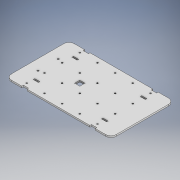
# Autodesk Inventor part: FPVchasisdraft2
Saved by Autodesk Inventor 2020 (Build 240168000, 168)
## iProperties
Created: 2020-11-26
Part Number: FPVchasisdraft2
Material: Generic
Document SubType Name: Modeling
Designer: yeyet
Density: 1 g/cm^3
Appearance: Default
Author: yeyet
Autodesk Inventor part; units mm, degrees
sketch "Sketch1" plane through (0, 0, 0) normal (0, 0, 1) x (1, 0, 0)
  line L0 (0, 0) -> (200, 0)
  line L1 (200, 0) -> (200, 120)
  line L2 (200, 120) -> (0, 120)
  line L3 (0, 120) -> (0, 0)
  dimension "d6" = 200
  dimension "d7" = 120
  constraints: 8 end point, 2 parallel, 1 horizontal, 1 perpendicular
  measures "d6" distance of L1.end L2.end
  measures "d7" distance of L0.end L1.end
extrude "Extrusion1" add sketch "Sketch1" along normal blind 3
sketch "Sketch2" plane through (0, 0, 3) normal (0, 0, 1) x (1, 0, 0)
  line L0 (0, 120) -> (0, 0) construction
  line L1 (0, 60) -> (200, 60) construction
  line L2 (200, 0) -> (200, 120) construction
  line L3 (200, 120) -> (0, 120) construction
  line L4 (100, 120) -> (100, 0) construction
  line L5 (0, 0) -> (200, 0) construction
  point P0 (30, 43.15)
  dimension "d10" = 16.85
  dimension "d11" = 30
  constraints: 4 end point, 4 midpoint
  measures "d10" distance from line of L1 point (30, 43.15)
  measures "d11" distance from line of point (30, 43.15) L0
hole "Hole1" at (30, 43.15, 3) direction (0, 0, -1) diameter 2.85 end through all thread size "M3.5x0.6" class "6H" standard "ISO Metric profile"
ref_plane "Work Plane1" through (0, 60, 0) normal (0, 1, 0) x (1, 0, 0)
mirror "Mirror1" about plane through (0, 60, 0) normal (0, 1, 0) of "Hole1"
pattern_linear "Rectangular Pattern1" count 2 spacing 33.7 along (1, 0, 0) of "Hole1", "Mirror1"
pattern_linear "Rectangular Pattern2" count 4 spacing 33.7 along (1, 0, 0) count 2 spacing 33.7 along (0, 1, 0) of "Hole1", "Mirror1", "Rectangular Pattern1"
mirror "Mirror2" about plane through (0, 60, 0) normal (0, 1, 0) of "Hole1", "Mirror1", "Rectangular Pattern1", "Rectangular Pattern2"
sketch "Sketch3" plane through (0, 0, 3) normal (0, 0, 1) x (1, 0, 0)
  line L0 (75.55, 65) -> (85.55, 65)
  line L1 (85.55, 65) -> (85.55, 55)
  line L2 (85.55, 55) -> (75.55, 55)
  line L3 (75.55, 55) -> (75.55, 65)
  circle A0 centre (63.7, 76.85) radius 1.425 construction
  circle A1 centre (97.4, 43.15) radius 1.425 construction
  line L4 (63.7, 76.85) -> (97.4, 43.15) construction
  circle A2 centre (97.4, 76.85) radius 1.425 construction
  circle A3 centre (63.7, 43.15) radius 1.425 construction
  line L5 (63.7, 43.15) -> (97.4, 76.85) construction
  point P0 (0, 0)
  point P1 (80.55, 65)
  point P2 (80.55, 60)
  point P3 (85.55, 60)
  point P4 (80.55, 60)
  dimension "d28" = 10
  dimension "d29" = 10
  constraints: 12 end point, 4 midpoint, 2 parallel, 1 horizontal, 1 horizontal alignment, 1 perpendicular, 1 vertical alignment
  measures "d28" distance of L0.end L1.end
  measures "d29" distance of L0.start L0.end
extrude "Extrusion2" cut sketch "Sketch3" against normal through all
sketch "Sketch4" plane through (0, 0, 3) normal (0, 0, 1) x (1, 0, 0)
  line L0 (0, 0) -> (200, 0) construction
  line L1 (30, 0) -> (40, 0)
  line L2 (40, 0) -> (40, 3)
  line L3 (40, 3) -> (30, 3)
  line L4 (30, 3) -> (30, 0)
  line L5 (0, 120) -> (0, 0) construction
  line L6 (30, 24.6) -> (40, 24.6)
  line L7 (40, 24.6) -> (40, 21.6)
  line L8 (40, 21.6) -> (30, 21.6)
  line L9 (30, 21.6) -> (30, 24.6)
  dimension "d32" = 3
  dimension "d33" = 10
  dimension "d34" = 30
  dimension "d35" = 18.6
  dimension "d36" = 3
  dimension "d37" = 10
  constraints: 16 end point, 4 parallel, 2 horizontal, 2 perpendicular, 2 point on line
  measures "d32" distance of L3.end L1.start
  measures "d33" distance of L2.end L3.end
  measures "d34" distance between parallel lines of L5 L4
  measures "d35" distance between parallel lines of L3 L8
  measures "d36" distance of L6.end L7.end
  measures "d37" distance of L6.start L6.end
extrude "Extrusion3" cut sketch "Sketch4" against normal through all
ref_plane "Work Plane66" through (0, 60, 0) normal (0, 1, 0) x (1, 0, 0)
mirror "Mirror3" about plane through (0, 60, 0) normal (0, 1, 0) of "Extrusion3"
ref_plane "Work Plane67" through (100, 0, 0) normal (-1, 0, 0) x (0, 0, 1)
mirror "Mirror4" about plane through (100, 0, 0) normal (-1, 0, 0) of "Extrusion3", "Mirror3"
sketch "Sketch5" plane through (0, 0, 3) normal (0, 0, 1) x (1, 0, 0)
  line L0 (0, 120) -> (0, 0) construction
  line L1 (0, 120) -> (0, 0) construction
  line L2 (0, 60) -> (200, 60) construction
  line L3 (200, 0) -> (200, 120) construction
  point P0 (20, 40.7)
  dimension "d40" = 20
  dimension "d41" = 19.3
  constraints: 2 end point, 2 midpoint
  measures "d40" distance from line of point (20, 40.7) L0
  measures "d41" distance from line of L2 point (20, 40.7)
hole "Hole2" at (20, 40.7, 3) direction (0, 0, -1) diameter 3.242 end through all thread size "M4x0.7" class "6H" standard "ISO Metric profile"
ref_plane "Work Plane68" through (40, 60, 0) normal (0, -1, 0) x (1, 0, 0)
mirror "Mirror5" about plane through (40, 60, 0) normal (0, -1, 0) of "Hole2"
fillet "Fillet1" radius 10 4 edges at (0, 120, 1.5) (0, 0, 1.5) (200, 0, 1.5) (200, 120, 1.5)
ref_plane "Work Plane2" through (0, 60, 0) normal (0, 1, 0) x (1, 0, 0)
ref_plane "Work Plane4" through (33.7, 60, 0) normal (0, 1, 0) x (1, 0, 0)
ref_plane "Work Plane5" through (33.7, 60, 0) normal (0, 1, 0) x (1, 0, 0)
ref_plane "Work Plane6" through (33.7, 60, 0) normal (0, 1, 0) x (1, 0, 0)
ref_plane "Work Plane7" through (67.4, 60, 0) normal (0, 1, 0) x (1, 0, 0)
ref_plane "Work Plane8" through (101.1, 60, 0) normal (0, 1, 0) x (1, 0, 0)
ref_plane "Work Plane9" through (0, 93.7, 0) normal (0, 1, 0) x (1, 0, 0)
ref_plane "Work Plane10" through (33.7, 93.7, 0) normal (0, 1, 0) x (1, 0, 0)
ref_plane "Work Plane11" through (67.4, 93.7, 0) normal (0, 1, 0) x (1, 0, 0)
ref_plane "Work Plane12" through (101.1, 93.7, 0) normal (0, 1, 0) x (1, 0, 0)
ref_plane "Work Plane13" through (33.7, 60, 0) normal (0, 1, 0) x (1, 0, 0)
ref_plane "Work Plane14" through (67.4, 60, 0) normal (0, 1, 0) x (1, 0, 0)
ref_plane "Work Plane15" through (101.1, 60, 0) normal (0, 1, 0) x (1, 0, 0)
ref_plane "Work Plane16" through (0, 93.7, 0) normal (0, 1, 0) x (1, 0, 0)
ref_plane "Work Plane17" through (33.7, 93.7, 0) normal (0, 1, 0) x (1, 0, 0)
ref_plane "Work Plane18" through (67.4, 93.7, 0) normal (0, 1, 0) x (1, 0, 0)
ref_plane "Work Plane19" through (101.1, 93.7, 0) normal (0, 1, 0) x (1, 0, 0)
ref_plane "Work Plane20" through (67.4, 60, 0) normal (0, 1, 0) x (1, 0, 0)
ref_plane "Work Plane21" through (101.1, 60, 0) normal (0, 1, 0) x (1, 0, 0)
ref_plane "Work Plane22" through (134.8, 60, 0) normal (0, 1, 0) x (1, 0, 0)
ref_plane "Work Plane23" through (33.7, 93.7, 0) normal (0, 1, 0) x (1, 0, 0)
ref_plane "Work Plane24" through (67.4, 93.7, 0) normal (0, 1, 0) x (1, 0, 0)
ref_plane "Work Plane25" through (101.1, 93.7, 0) normal (0, 1, 0) x (1, 0, 0)
ref_plane "Work Plane26" through (134.8, 93.7, 0) normal (0, 1, 0) x (1, 0, 0)
ref_plane "Work Plane27" through (67.4, 60, 0) normal (0, 1, 0) x (1, 0, 0)
ref_plane "Work Plane28" through (101.1, 60, 0) normal (0, 1, 0) x (1, 0, 0)
ref_plane "Work Plane29" through (134.8, 60, 0) normal (0, 1, 0) x (1, 0, 0)
ref_plane "Work Plane30" through (33.7, 93.7, 0) normal (0, 1, 0) x (1, 0, 0)
ref_plane "Work Plane31" through (67.4, 93.7, 0) normal (0, 1, 0) x (1, 0, 0)
ref_plane "Work Plane32" through (101.1, 93.7, 0) normal (0, 1, 0) x (1, 0, 0)
ref_plane "Work Plane33" through (134.8, 93.7, 0) normal (0, 1, 0) x (1, 0, 0)
ref_plane "Work Plane34" through (0, 60, 0) normal (0, 1, 0) x (1, 0, 0)
ref_plane "Work Plane35" through (0, 60, 0) normal (0, 1, 0) x (1, 0, 0)
ref_plane "Work Plane36" through (33.7, 60, 0) normal (0, 1, 0) x (1, 0, 0)
ref_plane "Work Plane37" through (33.7, 60, 0) normal (0, 1, 0) x (1, 0, 0)
ref_plane "Work Plane38" through (134.8, 26.3, 0) normal (0, 1, 0) x (1, 0, 0)
ref_plane "Work Plane39" through (101.1, 26.3, 0) normal (0, 1, 0) x (1, 0, 0)
ref_plane "Work Plane40" through (67.4, 26.3, 0) normal (0, 1, 0) x (1, 0, 0)
ref_plane "Work Plane41" through (33.7, 26.3, 0) normal (0, 1, 0) x (1, 0, 0)
ref_plane "Work Plane42" through (134.8, 60, 0) normal (0, 1, 0) x (1, 0, 0)
ref_plane "Work Plane43" through (101.1, 60, 0) normal (0, 1, 0) x (1, 0, 0)
ref_plane "Work Plane44" through (67.4, 60, 0) normal (0, 1, 0) x (1, 0, 0)
ref_plane "Work Plane45" through (134.8, 26.3, 0) normal (0, 1, 0) x (1, 0, 0)
ref_plane "Work Plane46" through (101.1, 26.3, 0) normal (0, 1, 0) x (1, 0, 0)
ref_plane "Work Plane47" through (67.4, 26.3, 0) normal (0, 1, 0) x (1, 0, 0)
ref_plane "Work Plane48" through (33.7, 26.3, 0) normal (0, 1, 0) x (1, 0, 0)
ref_plane "Work Plane49" through (134.8, 60, 0) normal (0, 1, 0) x (1, 0, 0)
ref_plane "Work Plane50" through (101.1, 60, 0) normal (0, 1, 0) x (1, 0, 0)
ref_plane "Work Plane51" through (67.4, 60, 0) normal (0, 1, 0) x (1, 0, 0)
ref_plane "Work Plane52" through (101.1, 26.3, 0) normal (0, 1, 0) x (1, 0, 0)
ref_plane "Work Plane53" through (67.4, 26.3, 0) normal (0, 1, 0) x (1, 0, 0)
ref_plane "Work Plane54" through (33.7, 26.3, 0) normal (0, 1, 0) x (1, 0, 0)
ref_plane "Work Plane55" through (0, 26.3, 0) normal (0, 1, 0) x (1, 0, 0)
ref_plane "Work Plane56" through (101.1, 60, 0) normal (0, 1, 0) x (1, 0, 0)
ref_plane "Work Plane57" through (67.4, 60, 0) normal (0, 1, 0) x (1, 0, 0)
ref_plane "Work Plane58" through (33.7, 60, 0) normal (0, 1, 0) x (1, 0, 0)
ref_plane "Work Plane59" through (101.1, 26.3, 0) normal (0, 1, 0) x (1, 0, 0)
ref_plane "Work Plane60" through (67.4, 26.3, 0) normal (0, 1, 0) x (1, 0, 0)
ref_plane "Work Plane61" through (33.7, 26.3, 0) normal (0, 1, 0) x (1, 0, 0)
ref_plane "Work Plane62" through (0, 26.3, 0) normal (0, 1, 0) x (1, 0, 0)
ref_plane "Work Plane63" through (101.1, 60, 0) normal (0, 1, 0) x (1, 0, 0)
ref_plane "Work Plane64" through (67.4, 60, 0) normal (0, 1, 0) x (1, 0, 0)
ref_plane "Work Plane65" through (33.7, 60, 0) normal (0, 1, 0) x (1, 0, 0)
equation "\"d36\" = d32"
equation "\"d37\" = d33"
body "Solid1"
